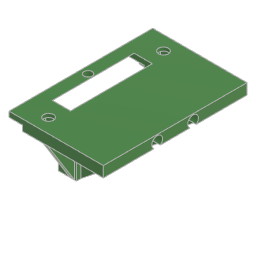
CR6_yaxis_assy (Autodesk Fusion 360 archive; units mm, degrees)
design "plate_bracket"
Autodesk Fusion 360 part; units mm, degrees
note: some values were not read from the file. Chosen so that the rebuilt part matches the saved one: a direction; which face or edge a step refers to. Set by a fixed rule: which sketch regions a step uses.
sketch "Sketch1" plane through (0, 0, 0) normal (1, 0, 0) x (0, 1, 0)
  line L0 (0, 0) -> (50, 0)
  line L1 (50, 0) -> (50, 30)
  line L2 (50, 30) -> (0, 30)
  line L3 (0, 30) -> (0, 0)
  dimension "d1" = 50
  dimension "d2" = 30
  constraint horizontal L0
  constraint vertical L1
  constraint horizontal L2
  constraint vertical L3
  constraint coincident L0.start L3.end
  measures "d1" distance of L0.start L0.end
  measures "d2" distance of L0.start L2.end
extrude "Extrude1" add sketch "Sketch1" along normal blind 10
sketch "Sketch2" plane through (0, 0, 0) normal (-1, 0, 0) x (0, -1, 0)
  line L0 (0, 0) -> (0, 30)
  line L1 (0, 30) -> (-50, 30)
  line L2 (-50, 30) -> (-50, 0)
  line L3 (-50, 0) -> (0, 0)
  line L4 (-25, 30) -> (-25, 0) construction
  line L5 (-47.75, 30) -> (-2.25, 30)
  line L6 (-2.25, 30) -> (-2.25, 2.9)
  line L7 (-2.25, 2.9) -> (-47.75, 2.9)
  line L8 (-47.75, 2.9) -> (-47.75, 30)
  line L9 (-25, 30) -> (-25, 2.9) construction
  line L10 (-15, 6.45) -> (-35, 6.45) construction
  line L11 (-35, 6.45) -> (-35, 26.45) construction
  line L12 (-35, 26.45) -> (-15, 26.45) construction
  line L13 (-15, 26.45) -> (-15, 6.45) construction
  line L14 (-15, 6.45) -> (-35, 26.45) construction
  line L15 (-35, 6.45) -> (-15, 26.45) construction
  point P0 (-25, 16.45)
  dimension "d5" = 27.1
  dimension "d6" = 45.5
  dimension "d7" = 20
  dimension "d8" = 20
  constraint midpoint L1 L4.start
  constraint midpoint L3 L4.end
  constraint horizontal L5
  constraint vertical L6
  constraint horizontal L7
  constraint vertical L8
  constraint coincident L1 L5.start
  constraint midpoint L5 L4.start
  constraint midpoint L7 L9.end
  constraint collinear L4 L9
  constraint horizontal L10
  constraint perpendicular L10 L11
  constraint parallel L10 L12
  constraint parallel L11 L13
  constraint coincident L14 P0
  constraint coincident L15 P0
  constraint midpoint L9 P0
  measures "d5" distance of L5.start L7.end
  measures "d6" distance of L6 L8
  measures "d7" distance of L11.end L12.end
  measures "d8" distance of L10.end L11.end
extrude "Extrude2" cut sketch "Sketch2" against normal blind 4.5 contours L1 L5 L6 L7 L8
hole "Hole1" at (0, 35, 26.45) at (0, 15, 6.45) at (0, 35, 6.45) at (0, 15, 26.45) direction (1, 0, 0) diameter 3.4 end through all
sketch "Sketch3" plane through (0, 0, 30) normal (0, 0, 1) x (-1, 0, 0)
  line L0 (0, -47.75) -> (-4.5, -47.75)
  line L1 (-4.5, -47.75) -> (-4.5, -2.25)
  line L2 (-4.5, -2.25) -> (0, -2.25)
  line L3 (0, -2.25) -> (0, 0)
  line L4 (0, 0) -> (-10, 0)
  line L5 (-10, 0) -> (-10, -50)
  line L6 (-10, -50) -> (0, -50)
  line L7 (0, -50) -> (0, -47.75)
  line L8 (-4.5, -47.75) -> (-4.5, -2.25)
  line L9 (-4.5, -2.25) -> (5.6, -2.25)
  line L10 (5.6, -2.25) -> (5.6, -47.75)
  line L11 (5.6, -47.75) -> (-4.5, -47.75)
  line L12 (-10, -25) -> (49, -25) construction
  line L13 (-10, -65) -> (12.5, -65)
  line L14 (12.5, -65) -> (12.5, 15)
  line L15 (12.5, 15) -> (-10, 15)
  line L16 (-10, 15) -> (-10, -65)
  line L17 (12.5, -25) -> (-10, -25) construction
  dimension "d14" = 10.1
  dimension "d15" = 22.5
  constraint perpendicular L8 L9
  constraint parallel L8 L10
  constraint parallel L9 L11
  constraint coincident L1.end L2.start
  constraint perpendicular L2 L8
  constraint coincident L0.end L1.start
  constraint midpoint L5 L12.start
  constraint perpendicular L5 L12
  constraint horizontal L13
  constraint vertical L14
  constraint horizontal L15
  constraint vertical L16
  constraint midpoint L14 L17.start
  constraint midpoint L16 L12.start
  constraint collinear L12 L17
  measures "d14" distance of L0.end L10.end
  measures "d15" distance of L13.start L13.end
extrude "Extrude3" add sketch "Sketch3" against normal blind 3 contours L3 L4 L6 L7 L9 L10 L11 L13 L14 L15 L16
sketch "Sketch4" plane through (0, 0, 27) normal (0, 0, -1) x (1, 0, 0)
  line L0 (10, -65) -> (10, -50)
  line L1 (10, -50) -> (0, -50)
  line L2 (0, -50) -> (0, -47.75)
  line L3 (0, -47.75) -> (-5.6, -47.75)
  line L4 (-5.6, -47.75) -> (-5.6, -2.25)
  line L5 (-5.6, -2.25) -> (0, -2.25)
  line L6 (0, -2.25) -> (0, 0)
  line L7 (0, 0) -> (10, 0)
  line L8 (10, 0) -> (10, 15)
  line L9 (10, 15) -> (-12.5, 15)
  line L10 (-12.5, 15) -> (-12.5, -65)
  line L11 (-12.5, -65) -> (10, -65)
  line L12 (10, 0) -> (-5, 0)
  line L13 (-5, 0) -> (-5, 15)
  line L14 (-5, 15) -> (10, 15)
  line L15 (10, 15) -> (10, 0)
  line L16 (10, -65) -> (-5, -65)
  line L17 (-5, -65) -> (-5, -50)
  line L18 (-5, -50) -> (10, -50)
  line L19 (10, -50) -> (10, -65)
  dimension "d31" = 15
  constraint horizontal L12
  constraint vertical L13
  constraint horizontal L14
  constraint vertical L15
  constraint coincident L9 L13.end
  constraint coincident L7.end L8.start
  constraint horizontal L16
  constraint vertical L17
  constraint horizontal L18
  constraint vertical L19
  constraint coincident L0.start L11.end
  measures "d31" distance of L13 L15
extrude "Extrude4" add sketch "Sketch4" along normal blind 3 contours L0 L1 L11 L16 L17 L18 L19 | L7 L8 L9 L12 L13 L14 L15
sketch "Sketch5" plane through (0, 0, 24) normal (0, 0, -1) x (1, 0, 0)
  line L0 (10, 15) -> (-5, 15)
  line L1 (-5, 15) -> (-5, 0)
  line L2 (0, 0) -> (10, 0)
  line L3 (10, 0) -> (10, 15)
  line L4 (1.5, 15) -> (1.5, -65) construction
  line L5 (5.425, 9.2661) -> (1.5, 11.5322)
  line L6 (1.5, 11.5322) -> (-2.425, 9.2661)
  line L7 (-2.425, 9.2661) -> (-2.425, 4.7339)
  line L8 (-2.425, 4.7339) -> (1.5, 2.4678)
  line L9 (1.5, 2.4678) -> (5.425, 4.7339)
  line L10 (5.425, 4.7339) -> (5.425, 9.2661)
  line L11 (5.425, -54.7339) -> (1.5, -52.4678)
  line L12 (1.5, -52.4678) -> (-2.425, -54.7339)
  line L13 (-2.425, -54.7339) -> (-2.425, -59.2661)
  line L14 (-2.425, -59.2661) -> (1.5, -61.5322)
  line L15 (1.5, -61.5322) -> (5.425, -59.2661)
  line L16 (5.425, -59.2661) -> (5.425, -54.7339)
  line L17 (-5, 0) -> (0, 0)
  point P0 (1.5, 7)
  point P1 (1.5, -57)
  point P2 (-8.5, -25)
  dimension "d21" = 8.5
  dimension "d22" = 3.925
  dimension "d23" = 3.925
  dimension "d24" = 64
  dimension "d25" = 8
  dimension "d32" = 32
  dimension "d33" = 10
  constraint coincident L0 L4.start
  constraint perpendicular L0 L4
  constraint coincident L4 P0
  constraint vertical L10
  constraint coincident L4 P1
  constraint vertical L16
  measures "d21" distance of L3 L4
  measures "d22" distance of P0 L10
  measures "d23" distance of P1 L16
  measures "d24" distance of P0 P1
  measures "d25" distance of L0 P0
  measures "d32" vertical distance of P0 P2
  measures "d33" horizontal distance of P0 P2
hole "Hole2" at (1.5, -7, 24) at (1.5, 57, 24) direction (0, 0, 1) diameter 5.5 depth 10 tip angle 118
extrude "Extrude5" cut sketch "Sketch5" against normal blind 4 contours L5 L6 L7 L8 L9 L10 | L11 L12 L13 L14 L15 L16
hole "Hole3" at (-8.5, 25, 24) direction (0, 0, 1) diameter 4.5 depth 10 tip angle 118
ref_plane "WorkPlane1" through (7.7125, -7, 26) normal (-1, 0, 0) x (0, -1, 0)
sketch "Sketch6" plane through (7.7125, -7, 26) normal (-1, 0, 0) x (0, 1, 0)
  line L0 (-8, 2) -> (7, 26)
  line L1 (57, 26) -> (72, 2)
rib "Rib1" add thickness 2.5 on both sides direction (0, 0.847998, 0.529999) up to next extending the curves path "Sketch6" along L0
rib "Rib2" add thickness 2.5 on both sides direction (0, -0.847998, 0.529999) up to next extending the curves path "Sketch6" along L1
chamfer "Chamfer1" distance 3 angle 45 1 edges at (-5.6, 25, 27)
chamfer "Chamfer2" distance 2.9 distance2 4.5 1 edges at (0, 25, 2.9) measured on face at (0, 17.4167, 0.9667)
sketch "Sketch7" plane through (10, 0, 0) normal (1, 0, 0) x (0, 1, 0)
  circle A0 centre (35, 6.45) radius 1.7
  circle A1 centre (35, 26.45) radius 1.7
  circle A2 centre (15, 6.45) radius 1.7
  circle A3 centre (15, 26.45) radius 1.7
  line L0 (0, 24) -> (0, 0)
  line L1 (0, 0) -> (50, 0)
  line L2 (50, 0) -> (50, 24)
  line L3 (50, 24) -> (65, 24)
  line L4 (65, 24) -> (65, 30)
  line L5 (65, 30) -> (-15, 30)
  line L6 (-15, 30) -> (-15, 24)
  line L7 (-15, 24) -> (0, 24)
  line L8 (25, 0) -> (25, 30) construction
  line L9 (-15, 30) -> (65, 30)
  line L10 (65, 30) -> (65, 24)
  line L11 (65, 24) -> (-15, 24)
  line L12 (-15, 24) -> (-15, 30)
  circle A4 centre (15, 26.45) radius 3
  circle A5 centre (35, 26.45) radius 3
  dimension "d45" = 6
  dimension "d46" = 6
  constraint midpoint L1 L8.start
  constraint midpoint L5 L8.end
  constraint horizontal L9
  constraint vertical L10
  constraint horizontal L11
  constraint vertical L12
  constraint coincident L5.end L6.start
  constraint collinear L4 L10
  constraint concentric A3 A4
  constraint concentric A1 A5
  measures "d45" diameter of A5
  measures "d46" diameter of A4
extrude "Extrude6" add sketch "Sketch7" along normal blind 30 contours L3 L4 L5 L6 L7 L9 L10 L11 L12 A4 A5
ref_plane "WorkPlane2" through (13.75, 5, 27) normal (0, -1, 0) x (-1, 0, 0)
ref_plane "WorkPlane3" through (13.75, 45, 27) normal (0, 1, 0) x (1, 0, 0)
ref_plane "WorkPlane4" through (13.75, 25, 27) normal (0, 1, 0) x (1, 0, 0)
sketch "Sketch8" plane through (10, 5, 27) normal (0, -1, 0) x (1, 0, 0)
  line L0 (0, -27) -> (30, -3)
sketch "Sketch9" plane through (10, 25, 27) normal (0, 1, 0) x (1, 0, 0)
  line L0 (0, 27) -> (30, 3)
sketch "Sketch10" plane through (10, 45, 27) normal (0, 1, 0) x (1, 0, 0)
  line L0 (0, 27) -> (30, 3)
rib "Rib3" add thickness 5 on both sides direction (-0.624695, 0, 0.780869) up to next extending the curves path "Sketch8" along L0
rib "Rib4" add thickness 5 on both sides direction (-0.624695, 0, 0.780869) up to next extending the curves path "Sketch9" along L0
rib "Rib5" add thickness 5 on both sides direction (-0.624695, 0, 0.780869) up to next extending the curves path "Sketch10" along L0
equation "d22 = ( 7.85 / 2 ) * 1 mm"
equation "d25 = ( ( 80 - 64 ) / 2 ) * 1 mm"

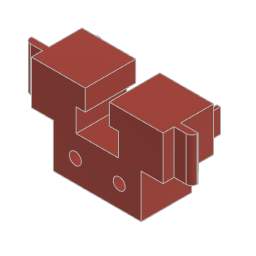
design "adapter"
Autodesk Fusion 360 part; units mm, degrees
sketch "Sketch1" plane through (0, 0, 0) normal (0, 1, 0) x (1, 0, 0)
  line L0 (0, 0) -> (0, -20) construction
  line L1 (0, -20) -> (30, -20)
  line L2 (30, -20) -> (30, 0)
  line L3 (30, 0) -> (20, 0)
  line L4 (20, 0) -> (20, 20)
  line L5 (20, 20) -> (0, 20)
  line L6 (-20, 0) -> (-20, 20)
  line L7 (-30, 0) -> (-20, 0)
  line L8 (-30, -20) -> (-30, 0)
  line L9 (-20, 20) -> (0, 20)
  line L10 (0, -20) -> (-30, -20)
  dimension "d1" = 20
  dimension "d2" = 30
  constraint coincident L0.start origin
  constraint vertical L0
  constraint perpendicular L0 L1
  constraint perpendicular L1 L2
  constraint perpendicular L2 L3
  constraint perpendicular L3 L4
  constraint perpendicular L4 L5
  constraint symmetric L1.start L0 L10.start
  constraint symmetric L0 L1.end L8.start
  constraint symmetric L0 L2.end L7.start
  constraint symmetric L0 L3.end L6.start
  constraint symmetric L0 L4.end L6.end
  constraint symmetric L0 L5.end L9.end
  measures "d1" distance of L0.start L0.end
  measures "d2" distance of L0.end L1.end
extrude "Extrude1" add sketch "Sketch1" along normal blind 15
sketch "Sketch2" plane through (0, 0, 0) normal (0, -1, 0) x (1, 0, 0)
  line L0 (30, 0) -> (30, 20)
  line L1 (30, 20) -> (-30, 20)
  line L2 (-30, 20) -> (-30, 0)
  line L3 (-30, 0) -> (-20, 0)
  line L4 (-20, 0) -> (-20, -20)
  line L5 (-20, -20) -> (20, -20)
  line L6 (20, -20) -> (20, 0)
  line L7 (20, 0) -> (30, 0)
  line L8 (30, 20) -> (38, 20)
  line L9 (38, 20) -> (38, 0)
  line L10 (38, 0) -> (30, 0)
  line L11 (30, 0) -> (30, 20)
  line L12 (-30, 20) -> (-38, 20)
  line L13 (-38, 20) -> (-38, 0)
  line L14 (-38, 0) -> (-30, 0)
  line L15 (-30, 0) -> (-30, 20)
  dimension "d5" = 8
  dimension "d6" = 8
  dimension "d7" = 20
  constraint horizontal L8
  constraint vertical L9
  constraint horizontal L10
  constraint vertical L11
  constraint coincident L0.end L1.start
  constraint horizontal L12
  constraint vertical L13
  constraint horizontal L14
  constraint vertical L15
  constraint coincident L1.end L2.start
  measures "d5" distance of L0.end L8.end
  measures "d6" distance of L1.end L12.end
  measures "d7" distance of L1.end L2.end
extrude "Extrude2" add sketch "Sketch2" along normal blind 3
sketch "Sketch3" plane through (0, -3, 0) normal (0, -1, 0) x (1, 0, 0)
  line L0 (38, 20) -> (-38, 20)
  line L1 (-38, 20) -> (-38, 0)
  line L2 (-38, 0) -> (-20, 0)
  line L3 (-20, 0) -> (-20, -20)
  line L4 (-20, -20) -> (20, -20)
  line L5 (20, -20) -> (20, 0)
  line L6 (20, 0) -> (38, 0)
  line L7 (38, 0) -> (38, 20)
  line L8 (-30, 20) -> (-30, 0)
  line L9 (0, 20) -> (-30, 20)
  line L10 (30, 20) -> (30, 0)
  line L11 (0, 20) -> (30, 20)
  line L12 (30, 0) -> (20, 0)
  line L13 (20, 0) -> (20, -20)
  line L14 (20, -20) -> (0, -20)
  line L15 (-20, -20) -> (0, -20)
  line L16 (-20, 0) -> (-20, -20)
  line L17 (-30, 0) -> (-20, 0)
extrude "Extrude3" add sketch "Sketch3" along normal blind 5 contours L0 L2 L3 L4 L5 L6 L8 L9 L10 L11 L12 L13 L14 L15 L16 L17
fillet "Fillet1" radius 2.5 2 edges at (38, -3, 10) (-38, -3, 10)
sketch "Sketch4" plane through (0, -8, 0) normal (0, -1, 0) x (1, 0, 0)
  line L0 (30, 20) -> (-30, 20)
  line L1 (-30, 20) -> (-30, 0)
  line L2 (-30, 0) -> (-20, 0)
  line L3 (-20, 0) -> (-20, -20)
  line L4 (-20, -20) -> (20, -20)
  line L5 (20, -20) -> (20, 0)
  line L6 (20, 0) -> (30, 0)
  line L7 (30, 0) -> (30, 20)
  line L8 (-20, -10) -> (20, -10) construction
  line L9 (20, 0) -> (20, -20)
  line L10 (-5.5, 20) -> (0, 20)
  line L11 (0, 20) -> (0, 13.9)
  line L12 (0, 13.9) -> (-5.5, 13.9)
  line L13 (-5.5, 13.9) -> (-5.5, 20)
  line L14 (0, 13.9) -> (5.5, 13.9)
  line L15 (5.5, 13.9) -> (5.5, 20)
  line L16 (5.5, 20) -> (0, 20)
  line L17 (14.8575, 20) -> (-15.1425, 20)
  line L18 (-15.1425, 20) -> (-15.1425, 10.5)
  line L19 (-15.1425, 10.5) -> (14.8575, 10.5)
  line L20 (14.8575, 10.5) -> (14.8575, 20)
  line L21 (14.8575, 20) -> (-15.1425, 10.5) construction
  line L22 (-15.1425, 20) -> (14.8575, 10.5) construction
  line L23 (9.65, 0) -> (-9.65, 0)
  line L24 (-9.65, 0) -> (-9.65, 10.5)
  line L25 (-9.65, 10.5) -> (9.65, 10.5)
  line L26 (9.65, 10.5) -> (9.65, 0)
  line L27 (9.65, 0) -> (-9.65, 10.5) construction
  line L28 (-9.65, 0) -> (9.65, 10.5) construction
  line L29 (5.5, 13.9) -> (14.8575, 13.9)
  line L30 (-15.1425, 13.9) -> (-5.5, 13.9)
  line L31 (-5.5, 13.9) -> (-5.5, 10.5)
  line L32 (5.5, 13.9) -> (5.5, 10.5)
  point P0 (-10, -10)
  point P1 (10, -10)
  point P2 (-0.1425, 15.25)
  point P3 (0, 5.25)
  dimension "d14" = 10
  dimension "d15" = 10
  dimension "d19" = 5.5
  dimension "d20" = 6.1
  dimension "d21" = 24.5
  dimension "d37" = 30
  dimension "d38" = 9.5
  dimension "d39" = 19.3
  dimension "d40" = 10.5
  constraint midpoint L3 L8.start
  constraint midpoint L5 L8.end
  constraint coincident L8 P0
  constraint coincident L8 P1
  constraint horizontal L10
  constraint vertical L11
  constraint horizontal L12
  constraint vertical L13
  constraint coincident L0 L10.start
  constraint symmetric L10.start L11 L15.end
  constraint symmetric L10.end L11 L16.end
  constraint symmetric L12.start L11 L14.start
  constraint symmetric L12.end L11 L14.end
  constraint horizontal L17
  constraint perpendicular L17 L18
  constraint parallel L17 L19
  constraint parallel L18 L20
  constraint coincident L21 P2
  constraint coincident L22 P2
  constraint collinear L0 L17
  constraint horizontal L23
  constraint perpendicular L23 L24
  constraint parallel L23 L25
  constraint parallel L24 L26
  constraint coincident L27 P3
  constraint coincident L28 P3
  constraint collinear L19 L25
  constraint coincident L20 L29.end
  constraint perpendicular L20 L29
  constraint coincident L18 L30.start
  constraint perpendicular L13 L30
  constraint coincident L25 L31.end
  constraint coincident L19 L32.end
  constraint vertical L32
  constraint vertical L31
  measures "d14" distance of L8.start P0
  measures "d15" distance of P1 L9
  measures "d19" distance of L11.end L12.end
  measures "d20" distance of L10.start L12.end
  measures "d21" distance of L0.end L13
  measures "d37" distance of L18.end L19.end
  measures "d38" distance of L17.end L18.end
  measures "d39" distance of L24.end L25.end
  measures "d40" distance of L23.end L24.end
hole "Hole1" at (10, -8, -10) at (-10, -8, -10) direction (0, 1, 0) diameter 5.5 end through all
extrude "Extrude4" cut sketch "Sketch4" against normal through all contours L0 L11 L14 L15 L16 L17 | L0 L10 L11 L12 L13 L17 | L12 L14 L19 L25 L31 L32 | L19 L23 L24 L25 L26
sketch "Sketch5" plane through (0, 15, 0) normal (0, 1, 0) x (-1, 0, 0)
  line L0 (-5.5, 20) -> (-30, 20)
  line L1 (-30, 20) -> (-30, 0)
  line L2 (-30, 0) -> (-20, 0)
  line L3 (-20, 0) -> (-20, -20)
  line L4 (-20, -20) -> (20, -20)
  line L5 (20, -20) -> (20, 0)
  line L6 (20, 0) -> (30, 0)
  line L7 (30, 0) -> (30, 20)
  line L8 (30, 20) -> (5.5, 20)
  circle A0 centre (-10, -10) radius 2.75
  circle A1 centre (10, -10) radius 2.75
  line L9 (0, 13.9) -> (0, -20) construction
  line L10 (-20, -10) -> (20, -10) construction
  line L11 (-16.55, -15.425) -> (-18.15, -15.425)
  line L12 (-18.15, -15.425) -> (-18.15, -4.575)
  line L13 (-18.15, -4.575) -> (-16.55, -4.575)
  line L14 (-16.55, -4.575) -> (-16.55, -15.425)
  line L15 (-16.55, -15.425) -> (-18.15, -4.575) construction
  line L16 (-18.15, -15.425) -> (-16.55, -4.575) construction
  line L17 (-13.95, -12.825) -> (-16.55, -12.825)
  line L18 (-16.55, -12.825) -> (-16.55, -7.175)
  line L19 (-16.55, -7.175) -> (-13.95, -7.175)
  line L20 (-13.95, -7.175) -> (-13.95, -12.825)
  line L21 (-13.95, -12.825) -> (-16.55, -7.175) construction
  line L22 (-16.55, -12.825) -> (-13.95, -7.175) construction
  line L23 (-16.55, -4.575) -> (-13.95, -7.175)
  line L24 (-13.95, -12.825) -> (-16.55, -15.425)
  line L25 (18.15, -4.575) -> (16.55, -4.575)
  line L26 (16.55, -4.575) -> (13.95, -7.175)
  line L27 (13.95, -7.175) -> (13.95, -12.825)
  line L28 (13.95, -12.825) -> (16.55, -15.425)
  line L29 (16.55, -15.425) -> (18.15, -15.425)
  line L30 (18.15, -15.425) -> (18.15, -4.575)
  line L31 (-30, 10) -> (30, 10) construction
  line L32 (-26.55, 4.575) -> (-28.15, 4.575)
  line L33 (-28.15, 4.575) -> (-28.15, 15.425)
  line L34 (-28.15, 15.425) -> (-26.55, 15.425)
  line L35 (-26.55, 15.425) -> (-26.55, 4.575)
  line L36 (-26.55, 4.575) -> (-28.15, 15.425) construction
  line L37 (-28.15, 4.575) -> (-26.55, 15.425) construction
  line L38 (-23.95, 7.175) -> (-26.55, 7.175)
  line L39 (-26.55, 7.175) -> (-26.55, 12.825)
  line L40 (-26.55, 12.825) -> (-23.95, 12.825)
  line L41 (-23.95, 12.825) -> (-23.95, 7.175)
  line L42 (-23.95, 7.175) -> (-26.55, 12.825) construction
  line L43 (-26.55, 7.175) -> (-23.95, 12.825) construction
  line L44 (-23.95, 12.825) -> (-26.55, 15.425)
  line L45 (-23.95, 7.175) -> (-26.55, 4.575)
  line L46 (23.95, 7.175) -> (26.55, 4.575)
  line L47 (23.95, 12.825) -> (23.95, 7.175)
  line L48 (23.95, 12.825) -> (26.55, 15.425)
  line L49 (28.15, 15.425) -> (26.55, 15.425)
  line L50 (28.15, 4.575) -> (28.15, 15.425)
  line L51 (26.55, 4.575) -> (28.15, 4.575)
  line L52 (5.5, 10.5) -> (9.65, 10.5)
  line L53 (9.65, 10.5) -> (9.65, 0)
  line L54 (9.65, 0) -> (-9.65, 0)
  line L55 (-9.65, 0) -> (-9.65, 10.5)
  line L56 (-9.65, 10.5) -> (-5.5, 10.5)
  line L57 (-5.5, 10.5) -> (-5.5, 20)
  line L58 (5.5, 20) -> (5.5, 10.5)
  point P0 (-17.35, -10)
  point P1 (-15.25, -10)
  point P2 (-27.35, 10)
  point P3 (-25.25, 10)
  dimension "d24" = 1.6
  dimension "d25" = 10.85
  dimension "d26" = 1.85
  dimension "d28" = 5.65
  dimension "d31" = 45
  dimension "d32" = 1.6
  dimension "d33" = 10.85
  dimension "d34" = 5.65
  dimension "d35" = 45
  dimension "d36" = 1.85
  constraint midpoint L4 L9.end
  constraint midpoint L3 L10.start
  constraint midpoint L5 L10.end
  constraint horizontal L11
  constraint perpendicular L11 L12
  constraint parallel L11 L13
  constraint parallel L12 L14
  constraint coincident L15 P0
  constraint coincident L16 P0
  constraint coincident L10 P0
  constraint horizontal L17
  constraint perpendicular L17 L18
  constraint parallel L17 L19
  constraint parallel L18 L20
  constraint coincident L21 P1
  constraint coincident L22 P1
  constraint coincident L10 P1
  constraint collinear L14 L18
  constraint symmetric L9 L11.start L28.end
  constraint symmetric L9 L11.end L29.end
  constraint symmetric L9 L12.end L25.start
  constraint symmetric L9 L13.end L25.end
  constraint symmetric L9 L17.start L27.end
  constraint symmetric L9 L19.end L26.end
  constraint midpoint L1 L31.start
  constraint midpoint L7 L31.end
  constraint horizontal L32
  constraint perpendicular L32 L33
  constraint parallel L32 L34
  constraint parallel L33 L35
  constraint coincident L36 P2
  constraint coincident L37 P2
  constraint coincident L31 P2
  constraint horizontal L38
  constraint perpendicular L38 L39
  constraint parallel L38 L40
  constraint parallel L39 L41
  constraint coincident L42 P3
  constraint coincident L43 P3
  constraint coincident L31 P3
  constraint collinear L35 L39
  constraint symmetric L9 L32.start L46.end
  constraint symmetric L9 L32.end L50.start
  constraint symmetric L9 L33.end L49.start
  constraint symmetric L9 L34.end L48.end
  constraint symmetric L9 L38.start L46.start
  constraint symmetric L9 L40.end L47.start
  measures "d24" distance of L12.end L13.end
  measures "d25" distance of L11.end L12.end
  measures "d26" distance of L3 L12
  measures "d28" distance of L17.end L18.end
  measures "d31" angle of L14 L23
  measures "d32" distance of L33.end L34.end
  measures "d33" distance of L32.end L33.end
  measures "d34" distance of L38.end L39.end
  measures "d35" angle of L35 L44
  measures "d36" distance of L1 L33
extrude "Extrude5" add sketch "Sketch5" along normal blind 5 contours L11 L12 L13 L14 L18 | L14 L17 L24 | L14 L17 L18 L19 L20 | L14 L19 L23 | L25 L26 L27 L28 L29 L30 | L32 L33 L34 L35 L39 | L35 L38 L45 | L35 L38 L39 L40 L41 | L35 L40 L44 | L46 L47 L48 L49 L50 L51
